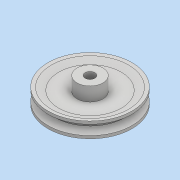
# Autodesk Inventor part: bánh đà
Saved by Autodesk Inventor 2018 (Build 220112000, 112)
## iProperties
Created: 2020-08-22
Part Number: bánh đà
Material: Generic
Document SubType Name: Modeling
Designer: ASUS
Density: 1 g/cm^3
Appearance: Default
Author: ASUS
Autodesk Inventor part; units mm, degrees
ref_plane "YZ Plane" through (0, 0, 0) normal (1, 0, 0) x (0, 1, 0)
ref_plane "XZ Plane" through (0, 0, 0) normal (0, 1, 0) x (-1, 0, 0)
ref_plane "XY Plane" through (0, 0, 0) normal (0, 0, 1) x (1, 0, 0)
sketch "Sketch1" plane through (0, 0, 0) normal (0, 1, 0) x (-1, 0, 0)
  line L0 (0.0054, 10.9523) -> (60.0054, 10.9523)
  line L1 (60.0054, 10.9523) -> (60.0054, -11.0477)
  line L2 (60.0054, -11.0477) -> (0.0054, -11.0477)
  line L3 (0.0054, -11.0477) -> (0.0054, 10.9523)
  line L4 (60.0054, 10.9523) -> (60.0054, 6.9523)
  line L5 (60.0054, -11.0477) -> (60.0054, -7.0477)
  line L6 (60.0054, -0.0477) -> (49.0054, -0.0477)
  line L7 (49, 3) -> (49, -3)
  line L8 (49, 3) -> (55, 3) construction
  line L9 (49, -3) -> (60.0054, -7.0477)
  line L10 (49, 3) -> (60.0054, 6.9523)
  line L11 (60.0054, 10.9523) -> (45.0054, 10.9523)
  line L12 (60.0054, 10.9523) -> (55.0244, 10.5165)
  line L13 (60.0054, 10.9523) -> (65.0054, 10.9523) construction
  line L14 (55.0244, 10.5165) -> (44.6878, 6.7543)
  line L15 (55.0244, 10.5165) -> (66.0244, 10.5165) construction
  line L16 (60.0054, -11.0477) -> (55.0244, -10.612)
  line L17 (60.0054, -11.0477) -> (65.0054, -11.0477) construction
  line L18 (55.0244, -10.612) -> (45.055, -5.9631)
  line L19 (0, 4) -> (0, -4)
  line L20 (0, 4) -> (8, 4) construction
  line L21 (0, -4) -> (45.055, -5.9631)
  line L22 (44.6878, 6.7543) -> (0, 4)
  dimension "d1" = 60
  dimension "d2" = 22
  dimension "d3" = 4
  dimension "d4" = 4
  dimension "d5" = 11
  dimension "d6" = 6
  dimension "d7" = 90
  dimension "d8" = 15
  dimension "d9" = 5
  dimension "d10" = 175
  dimension "d11" = 11
  dimension "d12" = 160
  dimension "d13" = 5
  dimension "d14" = 175
  dimension "d15" = 11
  dimension "d16" = 160
  dimension "d17" = 8
  dimension "d18" = 90
  constraints: 46 end point, 7 horizontal, 5 equal length, 3 parallel, 3 point on line, 1 midpoint, 1 perpendicular, 1 vertical
  measures "d1" distance of L1.end L2.end
  measures "d2" distance of L0.end L1.end
  measures "d3" distance of L0.end L4.end
  measures "d4" distance of L1.end L5.end
  measures "d5" distance of L6.start L6.end
  measures "d6" distance of L7.start L7.end
  measures "d7" angle of L7 L8
  measures "d8" distance of L0.end L11.end
  measures "d9" distance of L0.end L12.end
  measures "d10" angle of L12 L13
  measures "d11" distance of L12.end L14.end
  measures "d12" angle of L14 L15
  measures "d13" distance of L1.end L16.end
  measures "d14" angle of L17 L16
  measures "d15" distance of L16.end L18.end
  measures "d16" angle of L16 L18
  measures "d17" distance of L19.start L19.end
  measures "d18" angle of L19 L20
revolve "Revolution1" add sketch "Sketch1" angle 360 about axis through (0, 0, 4) along (0, 0, -1) contours L22 L14 L12 L1 L10 L7 L9 L16 L18 L21 L3 | L3 L21 L19 L22
sketch "Sketch2" plane through (0, 0, 0) normal (0, 0, 1) x (1, 0, 0)
  circle A0 centre (0, 0) radius 18.5
  dimension "d20" = 37
  constraints: 1 centre point, 1 coincident
  measures "d20" diameter of A0
extrude "Extrusion1" add sketch "Sketch2" along normal blind 25 and the other way blind 6
sketch "Sketch4" plane through (0, 0, 25) normal (0, 0, 1) x (1, 0, 0)
  circle A0 centre (0, 0) radius 7
  dimension "d25" = 14
  constraints: 1 centre point, 1 coincident
  measures "d25" diameter of A0
extrude "Extrusion2" cut sketch "Sketch4" against normal blind 36
body "Solid1"
